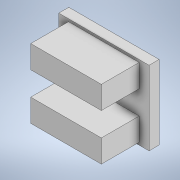
# Autodesk Inventor part: HDMI_Jumper
Saved by Autodesk Inventor 2021 (Build 250183000, 183)
## iProperties
Created: 2021-04-23
Part Number: HDMI_Jumper
Material: Generic
Document SubType Name: Modeling
Designer: trent
Density: 1 g/cm^3
Appearance: Default
Author: trent
Autodesk Inventor part; units mm, degrees
ref_plane "YZ Plane" through (0, 0, 0) normal (1, 0, 0) x (0, 1, 0)
ref_plane "XZ Plane" through (0, 0, 0) normal (0, 1, 0) x (-1, 0, 0)
ref_plane "XY Plane" through (0, 0, 0) normal (0, 0, 1) x (1, 0, 0)
sketch "Sketch1" plane through (0, 0, 0) normal (0, 0, 1) x (1, 0, 0)
  line L0 (0, 0) -> (17.9, 0)
  line L1 (17.9, 0) -> (17.9, 14.7)
  line L2 (17.9, 14.7) -> (0, 14.7)
  line L3 (0, 14.7) -> (0, 0)
  dimension "d0" = 17.9
  dimension "d1" = 14.7
  constraints: 8 end point, 2 parallel, 1 horizontal, 1 perpendicular
  measures "d0" distance of L1.end L2.end
  measures "d1" distance of L0.end L1.end
extrude "Extrusion1" add sketch "Sketch1" along normal blind 2
sketch "Sketch2" plane through (0, 0, 2) normal (0, 0, 1) x (1, 0, 0)
  line L0 (1.95, 0.5) -> (15.95, 0.5)
  line L1 (15.95, 0.5) -> (15.95, 5)
  line L2 (15.95, 5) -> (1.95, 5)
  line L3 (1.95, 5) -> (1.95, 0.5)
  line L4 (0, 0) -> (17.9, 0) projected
  line L5 (17.9, 0) -> (17.9, 14.7) projected
  line L6 (0, 14.7) -> (0, 0) projected
  line L7 (1.95, 9.7) -> (15.95, 9.7)
  line L8 (15.95, 9.7) -> (15.95, 14.2)
  line L9 (15.95, 14.2) -> (1.95, 14.2)
  line L10 (1.95, 14.2) -> (1.95, 9.7)
  line L11 (17.9, 14.7) -> (0, 14.7) projected
  dimension "d6" = 0.5
  dimension "d7" = 4.5
  dimension "d8" = 14
  dimension "d9" = 1.95
  dimension "d10" = 1.95
  dimension "d11" = 4.5
  dimension "d12" = 14
  dimension "d13" = 0.5
  dimension "d14" = 1.95
  dimension "d15" = 1.95
  constraints: 16 end point, 4 parallel, 2 horizontal, 2 perpendicular
  measures "d6" distance between parallel lines of L4 L0
  measures "d7" distance between parallel lines of L0 L2
  measures "d8" distance of L1.end L2.end
  measures "d9" distance between parallel lines of L5 L1
  measures "d10" distance between parallel lines of L6 L3
  measures "d11" distance between parallel lines of L7 L9
  measures "d12" distance of L8.end L9.end
  measures "d13" distance between parallel lines of L11 L9
  measures "d14" distance between parallel lines of L5 L8
  measures "d15" distance between parallel lines of L6 L10
extrude "Extrusion2" add sketch "Sketch2" along normal blind 7.5 contours L3 L2 L1 L0 | L10 L9 L8 L7
body "Solid1"
